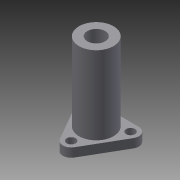
# Autodesk Inventor part: ScrewShaft
Saved by Autodesk Inventor 2013 (Build 170138000, 138)
## iProperties
Created: 2013-10-12
Part Number: ScrewShaft
Material: Generic
Document SubType Name: Modeling
Designer: cobrooks
Density: 1 g/cm^3
Author: cobrooks
Autodesk Inventor part; units mm, degrees
ref_plane "YZ Plane" through (0, 0, 0) normal (1, 0, 0) x (0, 1, 0)
ref_plane "XZ Plane" through (0, 0, 0) normal (0, 1, 0) x (-1, 0, 0)
ref_plane "XY Plane" through (0, 0, 0) normal (0, 0, 1) x (1, 0, 0)
sketch "Sketch1" plane through (0, 0, 0) normal (0, 1, 0) x (-1, 0, 0)
  circle A0 centre (0, 0) radius 9.8425
  circle A1 centre (0, 0) radius 5.08
  dimension "d0" = 19.685
  dimension "d1" = 10.16
  constraints: 2 centre point, 2 coincident
  measures "d0" diameter of A0
  measures "d1" diameter of A1
extrude "Extrusion1" add sketch "Sketch1" along normal blind 44.45
sketch "Sketch2" plane through (0, 0, 0) normal (0, -1, 0) x (1, 0, 0)
  circle A0 centre (0, 0) radius 9.8425 projected
  line L0 (4.0695, 16.6582) -> (16.4611, -4.8048)
  line L1 (12.3917, -11.8533) -> (-12.3917, -11.8533)
  line L2 (-16.4611, -4.8048) -> (-4.0695, 16.6582)
  arc A1 (4.0695, 16.6582) -> (-4.0695, 16.6582) centre (0, 14.3087) ccw
  arc A2 (-16.4611, -4.8048) -> (-12.3917, -11.8533) centre (-12.3917, -7.1543) ccw
  arc A3 (12.3917, -11.8533) -> (16.4611, -4.8048) centre (12.3917, -7.1543) ccw
  circle A4 centre (0, 0) radius 5.08 projected
  circle A5 centre (0, 0) radius 5.08
  point P0 (0, 23.7067)
  point P1 (20.5306, -11.8533)
  point P2 (-20.5306, -11.8533)
  dimension "d4" = 35.56
  dimension "d5" = 35.56
  dimension "d6" = 4.699
  dimension "d7" = 4.699
  dimension "d8" = 4.699
  constraints: 6 end point, 6 point on circle, 6 point on line, 6 tangent, 4 centre point, 2 coincident, 1 concentric, 7 other
  measures "d4" vertical distance of point (0, 23.707) point (20.531, -11.853)
  measures "d5" distance from line of point (0, 23.707) L1
  measures "d6" radius of A1
  measures "d7" radius of A2
  measures "d8" radius of A3
extrude "Extrusion2" add sketch "Sketch2" along normal blind 5.08 contours A0 | L0 A3 L1 A2 L2 A1
sketch "Sketch3" plane through (0, -5.08, 0) normal (0, -1, 0) x (1, 0, 0)
  arc A0 (4.0695, 16.6582) -> (-4.0695, 16.6582) centre (0, 14.3087) ccw projected
  arc A1 (-16.4611, -4.8048) -> (-12.3917, -11.8533) centre (-12.3917, -7.1543) ccw projected
  arc A2 (12.3917, -11.8533) -> (16.4611, -4.8048) centre (12.3917, -7.1543) ccw projected
  circle A3 centre (0, 14.3087) radius 2.54
  circle A4 centre (12.3917, -7.1543) radius 2.54
  circle A5 centre (-12.3917, -7.1543) radius 2.54
  dimension "d11" = 5.08
  dimension "d12" = 5.08
  dimension "d13" = 5.08
  constraints: 3 centre point, 3 coincident
  measures "d11" diameter of A3
  measures "d12" diameter of A4
  measures "d13" diameter of A5
extrude "Extrusion3" cut sketch "Sketch3" against normal blind 5.08
body "Solid1"
